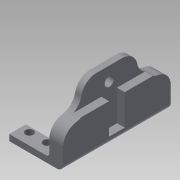
# Autodesk Inventor part: Pantilt
Saved by Autodesk Inventor 2013 (Build 170138000, 138)
## iProperties
Created: 2013-02-21
Part Number: Pantilt
Material: Générique
Document SubType Name: Modeling
Designer: UX31
Density: 1 g/cm^3
Author: UX31
Autodesk Inventor part; units mm, degrees
ref_plane "YZ Plane" through (0, 0, 0) normal (1, 0, 0) x (0, 1, 0)
ref_plane "XZ Plane" through (0, 0, 0) normal (0, 1, 0) x (-1, 0, 0)
ref_plane "XY Plane" through (0, 0, 0) normal (0, 0, 1) x (1, 0, 0)
sketch "Esquisse1" plane through (0, 0, 0) normal (0, 0, 1) x (1, 0, 0)
  line L0 (0, 0) -> (17.5, 0)
  line L1 (17.5, 0) -> (17.5, 35)
  line L2 (17.5, 35) -> (0, 35)
  line L3 (0, 35) -> (0, 0)
  dimension "d0" = 35
  dimension "d1" = 17.5
  constraints: 8 end point, 2 parallel, 1 horizontal, 1 perpendicular
  measures "d0" distance of L2.end L0.start
  measures "d1" distance of L1.end L2.end
extrude "Extrusion1" add sketch "Esquisse1" along normal blind 2
sketch "Esquisse2" plane through (0, 0, 2) normal (0, 0, 1) x (1, 0, 0)
  line L0 (0, 0) -> (17.5, 0) projected
  line L1 (17.5, 35) -> (0, 35) projected
  line L2 (0, 35) -> (0, 0) projected
  line L3 (0, 29.6) -> (11.43, 29.6)
  line L4 (11.43, 29.6) -> (11.43, 5.4)
  line L5 (11.43, 5.4) -> (0, 5.4)
  line L6 (0, 5.4) -> (0, 29.6)
  line L7 (11.43, 29.6) -> (11.43, 35) construction
  line L8 (11.43, 5.4) -> (11.43, 0) construction
  circle A0 centre (2.794, 31.25) radius 1.3
  circle A1 centre (8.636, 31.25) radius 1.3
  line L9 (11.43, 17.5) -> (0, 17.5) construction
  circle A2 centre (2.8364, 3.75) radius 1.3
  circle A3 centre (8.5936, 3.75) radius 1.3
  line L10 (8.5936, 3.75) -> (2.8364, 3.75) construction
  line L11 (8.636, 31.25) -> (2.794, 31.25) construction
  line L12 (5.715, 31.25) -> (5.715, 17.5) construction
  line L13 (5.715, 17.5) -> (5.715, 3.75) construction
  line L14 (2.794, 31.25) -> (0, 31.25) construction
  line L15 (8.636, 31.25) -> (11.43, 31.25) construction
  dimension "d4" = 24.2
  dimension "d6" = 11.43
  dimension "d7" = 5.842
  dimension "d8" = 27.5
  dimension "d9" = 2.6
  constraints: 26 end point, 5 collinear, 5 midpoint, 5 point on line, 4 centre point, 4 parallel, 4 perpendicular, 3 equal radius, 1 horizontal
  measures "d4" distance of L3.end L4.end
  measures "d6" distance of L3.start L3.end
  measures "d7" distance of L11.end L11.start
  measures "d8" distance between parallel lines of L10 L11
  measures "d9" diameter of A0
extrude "Extrusion2" cut sketch "Esquisse2" against normal blind 4.5
sketch "Esquisse3" plane through (0, 0, 2) normal (0, 0, 1) x (1, 0, 0)
  line L0 (0, 0) -> (17.5, 0) projected
  line L1 (17.5, 35) -> (13, 35)
  line L2 (13, 35) -> (13, 0)
  line L3 (13, 0) -> (17.5, 0)
  line L4 (17.5, 0) -> (17.5, 35)
  dimension "d12" = 4.5
  constraints: 8 end point, 2 parallel, 1 horizontal, 1 perpendicular, 1 point on line
  measures "d12" distance of L1.start L1.end
extrude "Extrusion3" add sketch "Esquisse3" along normal blind 10
sketch "Esquisse6" plane through (0, 0, 12) normal (0, 0, 1) x (1, 0, 0)
  line L0 (13, 0) -> (17.5, 0) construction
  line L1 (17.5, 0) -> (17.5, 35) construction
  line L2 (17.5, 35) -> (13, 35) construction
  line L3 (13, 35) -> (13, 0) construction
  line L4 (13, 26.5) -> (17.5, 26.5)
  line L5 (17.5, 26.5) -> (17.5, 8.5)
  line L6 (17.5, 8.5) -> (13, 8.5)
  line L7 (13, 8.5) -> (13, 26.5)
  line L8 (15.25, 26.5) -> (15.25, 35) construction
  line L9 (15.25, 8.5) -> (15.25, 0) construction
  point P0 (0, 0)
  dimension "d28" = 18
  constraints: 12 end point, 4 midpoint, 2 parallel, 2 point on line, 1 collinear, 1 horizontal, 1 perpendicular
  measures "d28" distance of L4.end L5.end
extrude "Extrusion6" add sketch "Esquisse6" along normal blind 8
fillet "Congé2" radius 5 2 edges at (15.25, 0, 12) (15.25, 35, 12)
fillet "Congé3" radius 5 4 edges at (15.25, 26.5, 12) (15.25, 8.5, 12) (15.25, 26.5, 20) (15.25, 8.5, 20)
sketch "Esquisse4" plane through (17.5, 0, 0) normal (1, 0, 0) x (0, 0, -1)
  line L0 (0, 0) -> (0, 35) construction
  line L1 (0, 35) -> (-12, 35) construction
  line L2 (0, 0) -> (-12, 0) construction
  line L3 (-27.5, 30.05) -> (-12.5, 30.05)
  line L4 (-12.5, 30.05) -> (-12.5, 20.05)
  line L5 (-12.5, 20.05) -> (-2.5, 20.05)
  line L6 (-2.5, 20.05) -> (-2.5, 14.95)
  line L7 (-2.5, 14.95) -> (-12.5, 14.95)
  line L8 (-12.5, 14.95) -> (-12.5, 4.95)
  line L9 (-12.5, 4.95) -> (-27.5, 4.95)
  line L10 (-27.5, 4.95) -> (-27.5, 30.05)
  line L11 (-7.5, 20.05) -> (-7.5, 35) construction
  line L12 (-7.5, 14.95) -> (-7.5, 0) construction
  dimension "d15" = 10
  dimension "d17" = 5.1
  dimension "d18" = 2.5
  dimension "d19" = 15
  constraints: 20 end point, 6 parallel, 4 equal length, 3 perpendicular, 2 midpoint, 2 point on line, 1 collinear
  measures "d15" distance of L4.end L5.end
  measures "d17" distance of L5.end L6.end
  measures "d18" distance between parallel lines of L0 L6
  measures "d19" distance of L3.start L3.end
extrude "Extrusion4" cut sketch "Esquisse4" against normal blind 2.5
sketch "Esquisse5" plane through (15, 0, 0) normal (1, 0, 0) x (0, 0, -1)
  line L0 (-12.5, 29.1009) -> (-12.5, 20.05) construction
  circle A0 centre (-15.5, 17.5) radius 1.5
  line L1 (-15.5, 17.5) -> (-12.5, 20.05) construction
  line L2 (-15.5, 17.5) -> (-12.5, 14.95) construction
  point P0 (-12.5, 4.95)
  point P1 (-12.5, 30.05)
  point P2 (0, 0)
  point P3 (-12.5, 29)
  dimension "d22" = 3
  dimension "d23" = 3
  constraints: 4 end point, 1 centre point, 1 equal length
  measures "d22" diameter of A0
  measures "d23" distance from line of L0 L1.start
extrude "Extrusion5" cut sketch "Esquisse5" against normal up to next
fillet "Congé1" radius 2 1 edges at (17.5, 17.5, 0)
fillet "Congé4" radius 1 1 edges at (13, 17.5, 2)
